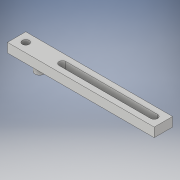
# Autodesk Inventor part: CameraSlider
Saved by Autodesk Inventor 2019 (Build 230136000, 136)
## iProperties
Created: 2019-07-15
Part Number: CameraSlider
Material: Generic
Document SubType Name: Modeling
Designer: aorfi
Density: 1 g/cm^3
Appearance: Default
Author: aorfi
Autodesk Inventor part; units mm, degrees
ref_plane "YZ Plane" through (0, 0, 0) normal (1, 0, 0) x (0, 1, 0)
ref_plane "XZ Plane" through (0, 0, 0) normal (0, 1, 0) x (-1, 0, 0)
ref_plane "XY Plane" through (0, 0, 0) normal (0, 0, 1) x (1, 0, 0)
sketch "Sketch1" plane through (0, 0, 0) normal (0, 1, 0) x (-1, 0, 0)
  line L0 (-40, 5) -> (40, 5)
  line L1 (40, 5) -> (40, -5)
  line L2 (40, -5) -> (-40, -5)
  line L3 (-40, -5) -> (-40, 5)
  line L4 (-40, 5) -> (40, -5) construction
  line L5 (40, 5) -> (-40, -5) construction
  circle A0 centre (15, 0) radius 1.8986
  circle A1 centre (-35, 0) radius 1.8986
  line L6 (15, 1.8986) -> (-35, 1.8986)
  line L7 (-35, -1.8987) -> (15, -1.8987)
  point P0 (0, 0)
  point P1 (0, 0)
  point P2 (35, 0)
  point P3 (0, 0)
  dimension "d0" = 80
  dimension "d1" = 10
  dimension "d2" = 3.7973
  dimension "d3" = 3.7973
  dimension "d4" = 25
  dimension "d5" = 5
  dimension "d8" = 5
  constraints: 16 end point, 4 midpoint, 4 point on circle, 4 tangent, 2 centre point, 2 horizontal, 2 horizontal alignment, 2 parallel, 1 perpendicular
  measures "d0" distance of L1.end L2.end
  measures "d1" distance of L0.end L1.end
  measures "d2" diameter of A0
  measures "d3" diameter of A1
  measures "d4" distance from line of A0.centre L1
  measures "d5" distance from line of L3 A1.centre
  measures "d8" distance from line of L1 point (35, 0)
extrude "Extrusion1" add sketch "Sketch1" along normal mid plane 5
sketch "Sketch2" plane through (0, -2.5, 0) normal (0, -1, 0) x (1, 0, 0)
  line L0 (-40, 5) -> (-40, -5) projected
  point P0 (0, 0)
  point P1 (-35, 0)
  point P2 (-40, 0)
  dimension "d16" = 5
  constraints: 1 horizontal alignment, 1 midpoint
  measures "d16" distance from line of L0 point (-35, 0)
hole "Hole2" at (-35, -2.5, 0) direction (0, 1, 0) diameter 3.797 end through all clearance for "Flat Head Machine Screw (82)" size "#6" standard "Ansi Unified Screw Threads"
sketch "Sketch3" plane through (0, -2.5, 0) normal (0, -1, 0) x (1, 0, 0)
  circle A0 centre (-27.5, 0) radius 2.5
  line L0 (-40, 5) -> (-40, -5) projected
  circle A1 centre (-35, 0) radius 1.8985 projected
  point P0 (0, 0)
  point P1 (-40, 0)
  dimension "d24" = 5
  dimension "d26" = 7.5
  constraints: 1 centre point, 1 horizontal alignment, 1 midpoint
  measures "d24" diameter of A0
  measures "d26" distance of A0.centre A1.centre
extrude "Extrusion2" add sketch "Sketch3" along normal blind 5 contours A0
equation "\"d3\" = d2"
body "Solid1"
